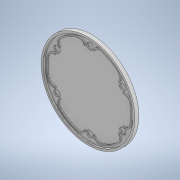
# Autodesk Inventor part: Bottom Lid
Saved by Autodesk Inventor 2020 (Build 240168000, 168)
## iProperties
Created: 2020-03-28
Part Number: Bottom Lid
Material: Generic
Document SubType Name: Modeling
Designer: pengpeng
Density: 1 g/cm^3
Appearance: Default
Author: pengpeng
Autodesk Inventor part; units mm, degrees
ref_plane "YZ Plane" through (0, 0, 0) normal (1, 0, 0) x (0, 1, 0)
ref_plane "XZ Plane" through (0, 0, 0) normal (0, 1, 0) x (-1, 0, 0)
ref_plane "XY Plane" through (0, 0, 0) normal (0, 0, 1) x (1, 0, 0)
sketch "Sketch3" plane through (0, 0, 0) normal (0, 0, 1) x (1, 0, 0)
  circle A0 centre (0, 0) radius 68
  circle A1 centre (0, 0) radius 65
  circle A2 centre (0, 0) radius 71
  dimension "d27" = 136
  dimension "d28" = 130
  dimension "d29" = 142
  constraints: 3 centre point, 3 coincident
  measures "d27" diameter of A0
  measures "d28" diameter of A1
  measures "d29" diameter of A2
extrude "Extrusion3" add sketch "Sketch3" along normal blind 3 contours A0 | A1 | A2
sketch "Sketch4" plane through (0, 0, 3) normal (0, 0, 1) x (1, 0, 0)
  circle A0 centre (0, 0) radius 71 projected
  line L0 (0, 0) -> (0, 63.1147) construction
  circle A1 centre (0, 57.5) radius 4.8
  circle A2 centre (-49.7965, 28.75) radius 4.8
  circle A3 centre (-49.7965, -28.75) radius 4.8
  circle A4 centre (0, -57.5) radius 4.8
  circle A5 centre (49.7965, -28.75) radius 4.8
  circle A6 centre (49.7965, 28.75) radius 4.8
  dimension "d32" = 9.6
  dimension "d33" = 57.5
  dimension "d36" = 360
  constraints: 6 centre point, 2 end point, 1 point on line, 1 vertical, 13 other
  measures "d32" diameter of A1
  measures "d33" distance of point (0, 0) A1.centre
extrude "Extrusion4" cut sketch "Sketch4" against normal blind 1.524 contours A1 | A2 | A3 | A4 | A5 | A6
sketch "Sketch5" plane through (0, 0, 3) normal (0, 0, 1) x (1, 0, 0)
  circle A0 centre (49.7965, -28.75) radius 4.8 projected
  circle A1 centre (-49.7965, 28.75) radius 4.8 projected
  circle A2 centre (49.7965, 28.75) radius 4.8 projected
  circle A3 centre (0, -57.5) radius 4.8 projected
  circle A4 centre (-49.7965, -28.75) radius 4.8 projected
  circle A5 centre (0, 57.5) radius 4.8 projected
  circle A6 centre (0, 0) radius 71 projected
  circle A7 centre (0, 57.5) radius 6.3
  circle A8 centre (-49.7965, 28.75) radius 6.3
  circle A9 centre (-49.7965, -28.75) radius 6.3
  circle A10 centre (0, -57.5) radius 6.3
  circle A11 centre (49.7965, -28.75) radius 6.3
  circle A12 centre (49.7965, 28.75) radius 6.3
  circle A13 centre (0, 0) radius 65
  circle A14 centre (-15.5907, 52.744) radius 10
  circle A15 centre (15.5907, 52.744) radius 10
  circle A16 centre (-37.8823, 39.874) radius 10
  circle A17 centre (-53.473, 12.87) radius 10
  circle A18 centre (-53.473, -12.87) radius 10
  circle A19 centre (-37.8823, -39.874) radius 10
  circle A20 centre (-15.5907, -52.744) radius 10
  circle A21 centre (15.5907, -52.744) radius 10
  circle A22 centre (37.8823, -39.874) radius 10
  circle A23 centre (53.473, -12.87) radius 10
  circle A24 centre (53.473, 12.87) radius 10
  circle A25 centre (37.8823, 39.874) radius 10
  circle A26 centre (-15.5907, 52.744) radius 8.5
  circle A27 centre (-37.8823, 39.874) radius 8.5
  arc A28 (-18.0002, 60.8953) -> (-43.7368, 46.0363) centre (0, 0) ccw
  line L0 (-45.1916, 33.0494) -> (-44.0952, 34.0731)
  line L1 (-6.0259, 55.6618) -> (-7.4606, 55.2241)
  line L2 (-51.2175, 22.6123) -> (-51.5558, 21.151)
  arc A29 (-61.737, 14.859) -> (-61.737, -14.859) centre (0, 0) ccw
  line L3 (-51.2175, -22.6123) -> (-51.5558, -21.151)
  circle A30 centre (-53.473, -12.87) radius 8.5
  circle A31 centre (-53.473, 12.87) radius 8.5
  line L4 (-45.1916, -33.0494) -> (-44.0952, -34.0731)
  arc A32 (-43.7368, -46.0363) -> (-18.0002, -60.8953) centre (0, 0) ccw
  line L5 (-6.0259, -55.6618) -> (-7.4606, -55.2241)
  circle A33 centre (-15.5907, -52.744) radius 8.5
  circle A34 centre (-37.8823, -39.874) radius 8.5
  line L6 (6.0259, -55.6618) -> (7.4606, -55.2241)
  arc A35 (18.0002, -60.8953) -> (43.7368, -46.0363) centre (0, 0) ccw
  line L7 (45.1916, -33.0494) -> (44.0952, -34.0731)
  circle A36 centre (37.8823, -39.874) radius 8.5
  circle A37 centre (15.5907, -52.744) radius 8.5
  line L8 (51.2175, -22.6123) -> (51.5558, -21.151)
  arc A38 (61.737, -14.859) -> (61.737, 14.859) centre (0, 0) ccw
  line L9 (51.2175, 22.6123) -> (51.5558, 21.151)
  circle A39 centre (53.473, 12.87) radius 8.5
  circle A40 centre (53.473, -12.87) radius 8.5
  line L10 (45.1916, 33.0494) -> (44.0952, 34.0731)
  arc A41 (43.7368, 46.0363) -> (18.0002, 60.8953) centre (0, 0) ccw
  line L11 (6.0259, 55.6618) -> (7.4606, 55.2241)
  circle A42 centre (15.5907, 52.744) radius 8.5
  circle A43 centre (37.8823, 39.874) radius 8.5
  point P0 (-63.1954, 15.2101)
  point P1 (-63.1954, -15.2101)
  point P2 (-45.1916, -33.0494)
  point P3 (-44.77, -47.1238)
  point P4 (-18.4254, -62.3338)
  point P5 (-6.0259, -55.6618)
  point P6 (6.0259, -55.6618)
  point P7 (18.4254, -62.3338)
  point P8 (44.77, -47.1238)
  point P9 (45.1916, -33.0494)
  point P10 (63.1954, -15.2101)
  point P11 (63.1954, 15.2101)
  point P12 (51.2175, 22.6123)
  point P13 (45.1916, 33.0494)
  point P14 (44.77, 47.1238)
  point P15 (18.4254, 62.3338)
  point P16 (6.0259, 55.6618)
  point P17 (-18.4254, 62.3338)
  point P18 (-44.77, 47.1238)
  dimension "d46" = 20
  dimension "d40" = 1.5
  dimension "d43" = 360
  dimension "d45" = 130
  dimension "d47" = 20
  dimension "d50" = 360
  dimension "d52" = 1.5
  dimension "d53" = 1.5
  dimension "d56" = 360
  constraints: 36 point on circle, 33 centre point, 24 end point, 2 coincident, 2 line through centre, 2 tangent, 137 other
  measures "d45" diameter of A13
  measures "d47" diameter of A15
extrude "Extrusion5" add sketch "Sketch5" along normal blind 1.5 contours L1 A26 A28 A14 | A15 A41 A42 L11 | A14 A28 A16 A13 | A13 A25 A41 A15 | A16 A28 A27 L0 | A25 L10 A43 A41 | A17 A29 A18 A13 | A17 L2 A31 A29 | A13 A23 A38 A24 | A24 A38 A39 L9 | A18 A29 A30 L3 | A19 A32 A20 A13 | A19 L4 A34 A32 | A23 L8 A40 A38 | A20 A32 A33 L5 | A13 A21 A35 A22 | A22 A35 A36 L7 | A21 L6 A37 A35 picked at (-10.8394, 60.9083) picked at (10.8394, 60.9083) picked at (-44.9035, 46.1933) picked at (47.256, 41.1158) picked at (-62.4563, 15.7909) picked at (62.2412, 16.3841) picked at (-62.2412, -16.3841) picked at (-45.2691, -33.9863) picked at (62.4563, -15.7909) picked at (-10.8394, -60.9083) picked at (44.8652, -46.2495) picked at (10.8394, -60.9083)
sketch "Sketch6" plane through (0, 0, 3) normal (0, 0, 1) x (1, 0, 0)
  circle A0 centre (0, 0) radius 71 projected
  circle A1 centre (0, 0) radius 68
  dimension "d60" = 136
  constraints: 1 centre point, 1 coincident
  measures "d60" diameter of A1
extrude "Extrusion6" add sketch "Sketch6" along normal blind 3
equation "\"d47\" = d46"
equation "\"d53\" = d52"
body "Solid2"
